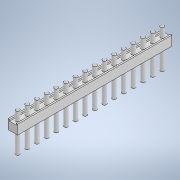
# Autodesk Inventor part: Гребенка 20 ПАПА
Saved by Autodesk Inventor 2020 (Build 240168000, 168)
## iProperties
Created: 2021-08-09
Part Number: Гребенка 20 ПАПА
Material: Типовые
Document SubType Name: Modeling
Designer: Антон
Density: 1 g/cm^3
Appearance: По умолчанию
Author: Антон
Autodesk Inventor part; units mm, degrees
ref_plane "YZ Plane" through (0, 0, 0) normal (1, 0, 0) x (0, 1, 0)
ref_plane "XZ Plane" through (0, 0, 0) normal (0, 1, 0) x (-1, 0, 0)
sketch "Эскиз1" plane through (0, 0, 0) normal (0, 1, 0) x (-1, 0, 0)
  circle A0 centre (0, 0) radius 0.5
  dimension "d0" = 1
  constraints: 1 centre point, 1 coincident
  measures "d0" diameter of A0
extrude "Выдавливание1" add sketch "Эскиз1" along normal blind 11
ref_plane "РабПлоскость1" through (0, 6, 0) normal (0, -1, 0) x (1, 0, 0)
sketch "Эскиз2" plane through (0, 6, 0) normal (0, -1, 0) x (1, 0, 0)
  circle A0 centre (0, 0) radius 0.5 projected
  line L0 (1.27, 1.27) -> (-1.27, 1.27)
  line L1 (-1.27, 1.27) -> (-1.27, -1.27)
  line L2 (-1.27, -1.27) -> (1.27, -1.27)
  line L3 (1.27, -1.27) -> (1.27, 1.27)
  line L4 (1.27, 1.27) -> (-1.27, -1.27) construction
  line L5 (-1.27, 1.27) -> (1.27, -1.27) construction
  dimension "d7" = 2.54
  dimension "d8" = 2.54
  constraints: 12 end point, 2 midpoint, 2 parallel, 1 horizontal, 1 perpendicular
  measures "d7" distance of L2.end L1.end
  measures "d8" distance of L1.end L0.end
extrude "Выдавливание2" add sketch "Эскиз2" against normal blind 2.5
sketch "Эскиз3" plane through (0, 8.5, 0) normal (0, 1, 0) x (1, 0, 0)
  line L0 (-0.87, -1.27) -> (0.87, -1.27)
  line L1 (0.87, -1.27) -> (0.87, 1.27)
  line L2 (0.87, 1.27) -> (-0.87, 1.27)
  line L3 (-0.87, 1.27) -> (-0.87, -1.27)
  circle A0 centre (0, 0) radius 0.5 projected
  line L4 (-0.87, -1.27) -> (0.87, 1.27) construction
  line L5 (0.87, -1.27) -> (-0.87, 1.27) construction
  line L6 (-1.27, -1.27) -> (1.27, -1.27) projected
  dimension "d11" = 1.74
  constraints: 12 end point, 2 midpoint, 2 parallel, 1 collinear, 1 horizontal, 1 perpendicular
  measures "d11" distance of L2.end L1.end
extrude "Выдавливание3" cut sketch "Эскиз3" against normal blind 0.4
chamfer "Фаска1" distance 0.5 angle 45 2 edges at (0.5, 11, 0) (0.5, 0, 0)
pattern_linear "Прямоуг.массив1" count 16 spacing 2.54 along (0, 0, -1) of "Выдавливание1", "Выдавливание2", "Выдавливание3", "Фаска1"
